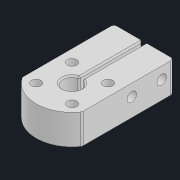
# Autodesk Inventor part: s_base3
Saved by Autodesk Inventor 2021 (Build 250183000, 183)
## iProperties
Created: 2021-08-20
Part Number: s_base3
Material: 一般
Document SubType Name: Modeling
Designer: yuta0
Density: 1 g/cm^3
Appearance: 既定
Author: yuta0
Autodesk Inventor part; units mm, degrees
ref_plane "YZ Plane" through (0, 0, 0) normal (1, 0, 0) x (0, 1, 0)
ref_plane "XZ Plane" through (0, 0, 0) normal (0, 1, 0) x (-1, 0, 0)
ref_plane "XY Plane" through (0, 0, 0) normal (0, 0, 1) x (1, 0, 0)
sketch "スケッチ1" plane through (0, 0, 0) normal (0, 1, 0) x (-1, 0, 0)
  line L0 (-10, 12) -> (10, 12)
  line L1 (10, 12) -> (10, -24)
  line L2 (10, -24) -> (-10, -24)
  line L3 (-10, -24) -> (-10, 12)
  circle A0 centre (0, 0) radius 12
  point P0 (10, 6.6332)
  point P1 (-10, 6.6332)
  dimension "d47" = 20
  dimension "d66" = 10
  dimension "d67" = 24
  dimension "d70" = 12
  constraints: 8 end point, 2 parallel, 1 centre point, 1 coincident, 1 horizontal, 1 perpendicular, 1 tangent
  measures "d47" distance of L0.start L0.end
  measures "d66" distance from line of point (0, 0) L1
  measures "d67" distance from line of point (0, 0) L2
  measures "d70" distance from line of point (0, 0) L0
extrude "押し出し1" add sketch "スケッチ1" along normal blind 10 contours A0 L1 L3 | A0 L1 L2 L3
sketch "スケッチ3" plane through (0, 10, 0) normal (0, 1, 0) x (1, 0, 0)
  circle A0 centre (0, 0) radius 8.5
  point P0 (-6.0104, 6.0104)
  point P1 (-6.0104, -6.0104)
  point P2 (6.0104, -6.0104)
  point P3 (6.0104, 6.0104)
  dimension "d6" = 17
  dimension "d9" = 360
  constraints: 1 coincident, 1 horizontal alignment, 8 other
hole "穴1" at (-6.0104, 10, -6.0104) at (-6.0104, 10, 6.0104) at (6.0104, 10, 6.0104) at (6.0104, 10, -6.0104) direction (0, -1, 0) diameter 3.2 end through all clearance for "Socket Head Cap Screw" size "M3" standard "Ansi Metric M Profile"
sketch "スケッチ2" plane through (0, 10, 0) normal (0, 1, 0) x (1, 0, 0)
  line L0 (-0.5, 0) -> (0.5, 0)
  line L1 (0.5, 0) -> (0.5, 24)
  line L2 (0.5, 24) -> (-0.5, 24)
  line L3 (-0.5, 24) -> (-0.5, 0)
  arc A0 (-10, -6.6332) -> (10, -6.6332) centre (0, 0) ccw projected
  line L4 (10, 24) -> (-10, 24) projected
  dimension "d3" = 1
  dimension "d71" = 0.5
  constraints: 8 end point, 2 parallel, 1 horizontal, 1 midpoint, 1 perpendicular, 1 point on line
  measures "d3" distance of L1.end L2.end
  measures "d71" distance from line of A0.centre L1
extrude "押し出し2" cut sketch "スケッチ2" against normal blind 8
sketch "スケッチ7" plane through (10, 0, 12) normal (1, 0, 0) x (0, 0, -1)
  line L0 (5.3668, 10) -> (36, 10) projected
  line L1 (36, 0) -> (36, 10) projected
  line L2 (12, -2) -> (12, 12) projected
  point P0 (12, 0)
  point P1 (22, 6)
  point P2 (32, 6)
  dimension "d48" = 4
  dimension "d50" = 4
  dimension "d68" = 10
  constraints: 1 horizontal alignment
  measures "d48" distance from line of L0 point (22, 6)
  measures "d50" distance from line of L1 point (32, 6)
  measures "d68" distance from line of L2 point (22, 6)
hole "穴4" at (10, 6, -10) at (10, 6, -20) direction (-1, 0, 0) diameter 3.2 end through all clearance for "Socket Head Cap Screw" size "M3" standard "Ansi Metric M Profile"
fillet "フィレット1" radius 1 4 edges at (10, 5, -24) (-10, 5, -24) (10, 5, 6.6332) (-10, 5, 6.6332)
sketch "スケッチ8" plane through (0, 0, 0) normal (0, -1, 0) x (1, 0, 0)
  circle A0 centre (0, 0) radius 3
  dimension "d62" = 6
  constraints: 1 centre point, 1 coincident
  measures "d62" diameter of A0
extrude "押し出し4" cut sketch "スケッチ8" against normal through all
chamfer "面取り2" distance 0.5 angle 45 10 edges at (-0.5, 10, -13.479) (0.5, 10, -13.479) (-1.9365, 10, 2.2913) (2.2913, 10, -1.9365) (-0.5, 6, -24) (0.5, 6, -24) (0, 2, -24) (0.5, 6, -2.958) (-0.5, 6, -2.958) (0, 2, -3)
equation "\"d66\" = 0.5 * d47"
equation "\"d50\" = d48"
